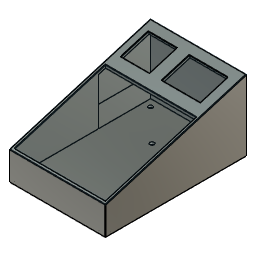
Macro pad v3 (Autodesk Fusion 360 design; units mm, degrees)
Autodesk Fusion 360 part; units mm, degrees
sketch "Esquisse1" plane through (0, 0, 0) normal (1, 0, 0) x (0, 1, 0)
  line L0 (-35, 0) -> (65, 0)
  line L1 (65, 0) -> (65, 50)
  line L2 (65, 50) -> (-35, 20)
  line L3 (-35, 20) -> (-35, 0)
  dimension "d1" = 20
  dimension "d2" = 100
  dimension "d3" = 50
  constraint horizontal L0
  constraint perpendicular L0 L1
  constraint perpendicular L0 L3
  measures "d1" distance of L0.start L2.end
  measures "d2" distance of L0.start L0.end
  measures "d3" distance of L0.end L1.end
extrude "Extrusion1" add sketch "Esquisse1" along normal blind 68
ref_plane "Plan de construction1" through (34, 15, 3) normal (0, 0, -1) x (0, 1, 0)
sketch "Esquisse2" plane through (0, 0, 3) normal (0, 0, -1) x (-1, 0, 0)
  line L0 (-2.0258, 31.0308) -> (-66.0258, 31.0308)
  line L1 (-66.0258, 31.0308) -> (-66.0258, -32.9692)
  line L2 (-66.0258, -32.9692) -> (-2.0258, -32.9692)
  line L3 (-2.0258, -32.9692) -> (-2.0258, 31.0308)
  dimension "d9" = 64
  dimension "d10" = 64
  constraint horizontal L0
  constraint vertical L1
  constraint horizontal L2
  constraint vertical L3
  measures "d9" distance of L0.start L0.end
  measures "d10" distance of L0.end L1.end
extrude "Extrusion2" cut sketch "Esquisse2" against normal blind 47
ref_plane "Plan de construction5" through (34, 15.5747, 33.0843) normal (0, -0.287348, 0.957826) x (0, -0.957826, -0.287348)
sketch "Esquisse3" plane through (0, -8.3945, 27.9817) normal (0, -0.287348, 0.957826) x (1, 0, 0)
  line L0 (2.0258, 41.1612) -> (66.0258, 41.1612)
  line L1 (66.0258, 41.1612) -> (66.0258, -25.6567)
  line L2 (66.0258, -25.6567) -> (2.0258, -25.6567)
  line L3 (2.0258, -25.6567) -> (2.0258, 41.1612)
  line L4 (0, 76.6261) -> (0, -27.777)
  line L5 (0, -27.777) -> (68, -27.777)
  line L6 (68, -27.777) -> (68, 76.6261)
  line L7 (68, 76.6261) -> (0, 76.6261)
sketch "Esquisse4" plane through (0, -7.8198, 26.066) normal (0, -0.287348, 0.957826) x (0, -0.957826, -0.287348)
ref_plane "Plan de construction7" through (34, 15, 3) normal (0, 0, -1) x (0, 1, 0)
sketch "Esquisse5" plane through (0, 0, 3) normal (0, 0, -1) x (-1, 0, 0)
  line L0 (-65.9985, 26.0001, 26.0687) -> (-1.9985, 26.0001, 26.0687)
  line L1 (-1.9985, 26.0001, 26.0687) -> (-1.9985, 63.0001, 26.0687)
  line L2 (-1.9985, 63.0001, 26.0687) -> (-65.9985, 63.0001, 26.0687)
  line L3 (-65.9985, 63.0001, 26.0687) -> (-65.9985, 26.0001, 26.0687)
  dimension "d21" = 64
  dimension "d22" = 37
extrude "Extrusion3" cut sketch "Esquisse5" against normal blind 15 from surface at -26.0687 contours L0 L1 L2 L3 in plane through (0, 0, -23.0687) normal (0, 0, -1)
ref_plane "Plan de construction11" through (34, 15, 3) normal (0, 0, -1) x (0, 1, 0)
sketch "Esquisse6" plane through (0, 0, 3) normal (0, 0, -1) x (-1, 0, 0)
  line L0 (-66.0001, 26) -> (-2.0001, 26)
  line L1 (-2.0001, 26) -> (-2.0001, 63)
  line L2 (-2.0001, 63) -> (-66.0001, 63)
  line L3 (-66.0001, 63) -> (-66.0001, 26)
  dimension "d28" = 37
  dimension "d29" = 64
  constraint horizontal L0
  constraint vertical L1
  constraint horizontal L2
  constraint vertical L3
  measures "d28" distance of L0.start L2.end
  measures "d29" distance of L1.end L2.end
extrude "Extrusion4" cut sketch "Esquisse6" along normal up to surface end surface through (34, 15.5747, 33.0843) normal (0, -0.287348, 0.957826) offset 0
fillet "Congé1" radius 0.3 12 edges at (0, 15, 35) (2.0258, -0.9692, 30.2092) (34.0258, 31.0308, 39.8092) (66.0258, -0.9692, 30.2092) (34.0258, -32.9692, 20.6092) (34, -35, 20) (68, 15, 35) (34, 65, 50) (0, -35, 10) (68, -35, 10) (68, 65, 25) (0, 65, 25)
sketch "Esquisse7" plane through (0, -8.3945, 27.9817) normal (0, -0.287348, 0.957826) x (1, 0, 0)
  line L0 (34, 69.6261) -> (61, 69.6261)
  line L1 (61, 69.6261) -> (61, 49.6261)
  line L2 (61, 49.6261) -> (34, 49.6261)
  line L3 (34, 49.6261) -> (34, 69.6261)
  line L4 (68, -27.777) -> (68, 76.6261)
  line L5 (68, 76.6261) -> (0, 76.6261)
  dimension "d35" = 20
  dimension "d36" = 7
  dimension "d37" = 7
  dimension "d38" = 27
  constraint horizontal L0
  constraint vertical L1
  constraint horizontal L2
  constraint vertical L3
  measures "d35" distance of L0.end L1.end
  measures "d36" distance of L1 L4
  measures "d37" distance of L0 L5
  measures "d38" distance of L1 L3
extrude "Extrusion5" cut sketch "Esquisse7" against normal blind 3
sketch "Esquisse8" plane through (0, -8.3945, 27.9817) normal (0, -0.287348, 0.957826) x (1, 0, 0)
  line L0 (5, 69.6261) -> (25, 69.6261)
  line L1 (25, 69.6261) -> (25, 49.6261)
  line L2 (25, 49.6261) -> (5, 49.6261)
  line L3 (5, 49.6261) -> (5, 69.6261)
  line L4 (68, 76.6261) -> (0, 76.6261)
  line L5 (0, 76.6261) -> (0, -27.777)
  dimension "d41" = 20
  dimension "d42" = 7
  dimension "d43" = 20
  dimension "d44" = 5
  constraint horizontal L0
  constraint vertical L1
  constraint horizontal L2
  constraint vertical L3
  measures "d41" distance of L0 L2
  measures "d42" distance of L0 L4
  measures "d43" distance of L1 L3
  measures "d44" distance of L3 L5
extrude "Extrusion6" cut sketch "Esquisse8" against normal blind 3
fillet "Congé2" radius 0.3 4 edges at (47.5, 58.2952, 47.9886) (61, 48.717, 45.1151) (47.5, 39.1387, 42.2416) (34, 48.717, 45.1151)
fillet "Congé3" radius 0.3 4 edges at (25, 48.717, 45.1151) (15, 39.1387, 42.2416) (15, 58.2952, 47.9886) (5, 48.717, 45.1151)
sketch "Esquisse9" plane through (0, 65, 0) normal (0, 1, 0) x (-1, 0, 0)
  line L0 (-0.3, 0) -> (-0.3, 49.5968)
  line L1 (-0.3, 49.5968) -> (-67.7, 49.5968)
  line L2 (-67.7, 49.5968) -> (-67.7, 0)
  line L3 (-67.7, 0) -> (-0.3, 0)
  line L4 (-57.7, 14) -> (-42.7, 14)
  line L5 (-42.7, 14) -> (-42.7, 4)
  line L6 (-42.7, 4) -> (-57.7, 4)
  line L7 (-57.7, 4) -> (-57.7, 14)
  dimension "d51" = 4
  dimension "d52" = 10
  dimension "d53" = 10
  dimension "d54" = 15
  constraint horizontal L4
  constraint vertical L5
  constraint horizontal L6
  constraint vertical L7
  measures "d51" distance of L3 L6
  measures "d52" distance of L2 L7
  measures "d53" distance of L4.end L5.end
  measures "d54" distance of L4.start L4.end
extrude "Extrusion7" cut sketch "Esquisse9" against normal blind 1 contours L4 L5 L6 L7
sketch "Esquisse10" plane through (0, 64, 0) normal (0, 1, 0) x (-1, 0, 0)
  line L0 (-57.7, 4) -> (-42.7, 4)
  line L1 (-42.7, 4) -> (-42.7, 14)
  line L2 (-42.7, 14) -> (-57.7, 14)
  line L3 (-57.7, 14) -> (-57.7, 4)
  line L4 (-55.2, 11.25) -> (-45.2, 11.25)
  line L5 (-45.2, 11.25) -> (-45.2, 6.75)
  line L6 (-45.2, 6.75) -> (-55.2, 6.75)
  line L7 (-55.2, 6.75) -> (-55.2, 11.25)
  dimension "d57" = 4.5
  dimension "d58" = 10
  dimension "d59" = 2.75
  dimension "d60" = 2.5
  constraint horizontal L4
  constraint vertical L5
  constraint horizontal L6
  constraint vertical L7
  measures "d57" distance of L4.end L5.end
  measures "d58" distance of L5.end L6.end
  measures "d59" distance of L0 L6
  measures "d60" distance of L3 L7
extrude "Extrusion8" cut sketch "Esquisse10" against normal blind 2 contours L4 L5 L6 L7
fillet "Congé4" radius 0.3 4 edges at (50.2, 65, 14) (57.7, 65, 9) (50.2, 65, 4) (42.7, 65, 9)
fillet "Congé5" radius 0.3 4 edges at (50.2, 63.0001, 6.75) (55.2, 64, 9) (50.2, 64, 11.25) (45.2, 64, 9)
ref_plane "Plan de construction12" through (34, 16.7241, 29.253) normal (0, -0.287348, 0.957826) x (1, 0, 0)
sketch "Esquisse11" plane through (0, -6.6704, 22.2347) normal (0, -0.287348, 0.957826) x (1, 0, 0)
ref_plane "Plan de construction13" through (34, 16.7241, 29.253) normal (0, -0.287348, 0.957826) x (1, 0, 0)
sketch "Esquisse12" plane through (0, -6.6704, 22.2347) normal (0, -0.287348, 0.957826) x (1, 0, 0)
ref_plane "Plan de construction14" through (34, 16.7241, 29.253) normal (0, -0.287348, 0.957826) x (1, 0, 0)
sketch "Esquisse13" plane through (0, -6.6704, 22.2347) normal (0, -0.287348, 0.957826) x (1, 0, 0)
sketch "Esquisse14" plane through (0, 0, 0) normal (0, 0, 1) x (1, 0, 0)
  circle A0 centre (4, -31) radius 3.5
  line L0 (0, -35) -> (68, -35)
  line L1 (0, 65) -> (0, -35)
  circle A1 centre (64, -31) radius 3.5
  line L2 (68, -35) -> (68, 65)
  circle A2 centre (7, 58) radius 3.5
  line L3 (68, 65) -> (0, 65)
  circle A3 centre (61, 58) radius 3.5
  point P0 (3.5, -31.5)
  dimension "d72" = 7
  dimension "d73" = 4
  dimension "d74" = 4
  dimension "d75" = 7
  dimension "d76" = 4
  dimension "d77" = 4
  dimension "d78" = 7
  dimension "d79" = 7
  dimension "d80" = 7
  dimension "d81" = 7
  dimension "d82" = 7
  dimension "d83" = 7
  measures "d72" diameter of A0
  measures "d73" distance of A0.centre L0
  measures "d74" distance of A0.centre L1
  measures "d75" diameter of A1
  measures "d76" distance of L0 A1.centre
  measures "d77" distance of A1.centre L2
  measures "d78" diameter of A2
  measures "d79" distance of A2.centre L3
  measures "d80" distance of L1 A2.centre
  measures "d81" diameter of A3
  measures "d82" distance of L3 A3.centre
  measures "d83" distance of L2 A3.centre
extrude "Extrusion9" cut sketch "Esquisse14" along normal blind 1.5 contours A0 | A1 | A2 | A3
sketch "Esquisse15" plane through (0, 0, 0) normal (0, 0, 1) x (1, 0, 0)
  circle A0 centre (30, 36) radius 3.5
  line L0 (68, 65) -> (0, 65)
  line L1 (68, -35) -> (68, 65)
  line L2 (0, 65) -> (0, -35)
  dimension "d86" = 7
  dimension "d87" = 29
  dimension "d89" = 30
  measures "d86" diameter of A0
  measures "d87" distance of A0.centre L0
  measures "d89" distance of A0.centre L2
extrude "Extrusion10" cut sketch "Esquisse15" along normal blind 1.5
sketch "Esquisse16" plane through (0, 0, 1.5) normal (0, 0, -1) x (1, 0, 0)
  circle A0 centre (61, -58) radius 3.5
  circle A1 centre (61, -58) radius 1.5
  dimension "d92" = 3
  constraint coincident A0.centre A1.centre
  measures "d92" diameter of A1
extrude "Extrusion11" cut sketch "Esquisse16" against normal blind 1.5 contours A1
sketch "Esquisse17" plane through (0, 0, 1.5) normal (0, 0, -1) x (1, 0, 0)
  circle A0 centre (7, -58) radius 3.5
  circle A1 centre (7, -58) radius 1.5
  dimension "d95" = 3
  constraint coincident A0.centre A1.centre
  measures "d95" diameter of A1
extrude "Extrusion12" cut sketch "Esquisse17" against normal blind 1.5 contours A1
sketch "Esquisse18" plane through (0, 0, 1.5) normal (0, 0, -1) x (1, 0, 0)
  circle A0 centre (30, -36) radius 3.5
  circle A1 centre (30, -36) radius 1.5
  dimension "d98" = 3
  constraint coincident A0.centre A1.centre
  measures "d98" diameter of A1
extrude "Extrusion13" cut sketch "Esquisse18" against normal blind 1.5 contours A1
sketch "Esquisse19" plane through (0, 0, 1.5) normal (0, 0, -1) x (1, 0, 0)
  circle A0 centre (64, 31) radius 3.5
  circle A1 centre (64, 31) radius 1.5
  dimension "d101" = 3
  constraint coincident A0.centre A1.centre
  measures "d101" diameter of A1
extrude "Extrusion14" cut sketch "Esquisse19" against normal blind 1.5 contours A1
sketch "Esquisse20" plane through (0, 0, 1.5) normal (0, 0, -1) x (1, 0, 0)
  circle A0 centre (4, 31) radius 3.5
  circle A1 centre (4, 31) radius 1.5
  dimension "d104" = 3
  constraint coincident A0.centre A1.centre
  measures "d104" diameter of A1
extrude "Extrusion15" cut sketch "Esquisse20" against normal blind 1.5 contours A1
